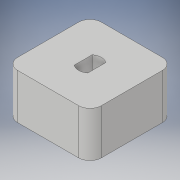
# Autodesk Inventor part: servo connector
Saved by Autodesk Inventor 2017 (Build 210142000, 142)
## iProperties
Created: 2017-01-19
Part Number: servo connector
Material: Generic
Document SubType Name: Modeling
Designer: Gabe Madonna
Density: 1 g/cm^3
Appearance: Default
Author: Gabe Madonna
Autodesk Inventor part; units mm, degrees
ref_plane "YZ Plane" through (0, 0, 0) normal (1, 0, 0) x (0, 1, 0)
ref_plane "XZ Plane" through (0, 0, 0) normal (0, 1, 0) x (-1, 0, 0)
ref_plane "XY Plane" through (0, 0, 0) normal (0, 0, 1) x (1, 0, 0)
sketch "Sketch1" plane through (0, 0, 0) normal (0, 1, 0) x (-1, 0, 0)
  line L0 (9.25, -9.25) -> (-9.25, -9.25)
  line L1 (-9.25, -9.25) -> (-9.25, 9.25)
  line L2 (-9.25, 9.25) -> (9.25, 9.25)
  line L3 (9.25, 9.25) -> (9.25, -9.25)
  point P0 (0, 0)
  point P1 (0, 0)
  dimension "d0" = 18.5
  constraints: 8 end point, 1 coincident, 9 other
  measures "d0" distance between parallel lines of L1 L3
extrude "Extrusion1" add sketch "Sketch1" along normal blind 10
fillet "Fillet1" radius 2.5 4 edges at (9.25, 5, 9.25) (-9.25, 5, 9.25) (9.25, 5, -9.25) (-9.25, 5, -9.25)
sketch "Sketch2" plane through (0, 10, 0) normal (0, 1, 0) x (1, 0, 0)
  circle A0 centre (0, 0) radius 2.5
  dimension "d4" = 5
  constraints: 1 centre point, 1 coincident
  measures "d4" diameter of A0
extrude "Extrusion2" cut sketch "Sketch2" against normal through all
sketch "Sketch3" plane through (0, 10, 0) normal (0, 1, 0) x (1, 0, 0)
  line L0 (-1.5, -2.5) -> (1.5, -2.5)
  line L1 (1.5, -2.5) -> (1.5, 2.5)
  line L2 (1.5, 2.5) -> (-1.5, 2.5)
  line L3 (-1.5, 2.5) -> (-1.5, -2.5)
  line L4 (-1.5, -2.5) -> (1.5, 2.5) construction
  line L5 (1.5, -2.5) -> (-1.5, 2.5) construction
  line L6 (-3.8508, -4.7625) -> (3.8508, -4.7625)
  line L7 (3.8508, -4.7625) -> (3.8508, 4.7625)
  line L8 (3.8508, 4.7625) -> (-3.8508, 4.7625)
  line L9 (-3.8508, 4.7625) -> (-3.8508, -4.7625)
  line L10 (-3.8508, -4.7625) -> (3.8508, 4.7625) construction
  line L11 (3.8508, -4.7625) -> (-3.8508, 4.7625) construction
  point P0 (0, 0)
  point P1 (0, 0)
  dimension "d7" = 3
  constraints: 24 end point, 4 midpoint, 4 parallel, 3 perpendicular, 1 horizontal
  measures "d7" distance of L0.start L0.end
extrude "Extrusion3" add sketch "Sketch3" against normal blind 7.5
body "Solid1"
